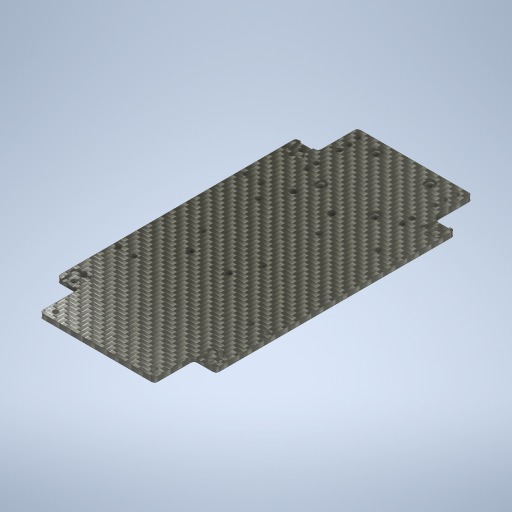
# Autodesk Inventor part: FootSoleFrame
Saved by Autodesk Inventor 2024.2 (Build 282272000, 272)
## iProperties
Created: 2024-01-07
Part Number: FootSoleFrame
Material: CFRP
Document SubType Name: Modeling
Designer: Masato Kubotera
Density: 1.43 g/cm^3
Appearance: Carbon Fiber 1
Mass: 79.1828 g
Surface Area: 392.308 cm^2
Volume: 55.3726 cm^3
Vendor: ALLPCB
Author: Masato Kubotera
Autodesk Inventor part; units mm, degrees
ref_plane "YZ Plane" through (0, 0, 0) normal (1, 0, 0) x (0, 1, 0)
ref_plane "XZ Plane" through (0, 0, 0) normal (0, 1, 0) x (-1, 0, 0)
ref_plane "XY Plane" through (0, 0, 0) normal (0, 0, 1) x (1, 0, 0)
sketch "Sketch1" plane through (0, 0, 0) normal (0, 0, 1) x (1, 0, 0)
  line L0 (-100, 59.95) -> (100, 59.95)
  line L1 (100, 59.95) -> (100, -40.05)
  line L2 (100, -40.05) -> (-100, -40.05)
  line L3 (-100, -40.05) -> (-100, 59.95)
  line L4 (-100, 59.95) -> (100, -40.05) construction
  line L5 (100, 59.95) -> (-100, -40.05) construction
  line L6 (0, -40.05) -> (0, 59.95) construction
  line L7 (-100, 9.95) -> (100, 9.95) construction
  line L8 (-100, 0) -> (100, 0) construction
  line L9 (-44, -22.5) -> (18, -22.5) construction
  line L10 (18, -22.5) -> (18, 22.5) construction
  line L11 (18, 22.5) -> (-44, 22.5) construction
  line L12 (-44, 22.5) -> (-44, -22.5) construction
  line L13 (-44, -22.5) -> (18, 22.5) construction
  line L14 (18, -22.5) -> (-44, 22.5) construction
  line L15 (13, -22.5) -> (13, 22.5) construction
  line L16 (4.5, -19) -> (4.5, 19) construction
  line L17 (-13, -22.5) -> (-13, 22.5) construction
  line L18 (-39, -22.5) -> (-39, 22.5) construction
  line L19 (100, 46.05) -> (75.15, 46.05)
  line L20 (75.15, 46.05) -> (75.15, 59.95)
  line L21 (65.2, 49.05) -> (97, 49.05) construction
  line L22 (97, 49.05) -> (97, 56.95) construction
  line L23 (97, 56.95) -> (65.2, 56.95) construction
  line L24 (65.2, 56.95) -> (65.2, 49.05) construction
  line L25 (65.2, 49.05) -> (97, 56.95) construction
  line L26 (97, 49.05) -> (65.2, 56.95) construction
  line L27 (65.2, 53) -> (97, 53) construction
  line L28 (81.1, 49.05) -> (81.1, 56.95) construction
  circle A0 centre (71.55, 53) radius 1.6 construction
  circle A1 centre (65.2, 53) radius 1.6 construction
  line L29 (100, -26.15) -> (75.15, -26.15)
  line L30 (75.15, -26.15) -> (75.15, -40.05)
  line L31 (-100, 46.05) -> (-75.15, 46.05)
  line L32 (-75.15, 46.05) -> (-75.15, 59.95)
  line L33 (-75.15, -26.15) -> (-75.15, -40.05)
  line L34 (-100, -26.15) -> (-75.15, -26.15)
  line L35 (13, -12) -> (18, -12) construction
  line L36 (13, 12) -> (18, 12) construction
  circle A2 centre (95, 41.05) radius 5 construction
  circle A3 centre (95, 41.05) radius 2 construction
  circle A4 centre (95, -21.15) radius 5 construction
  circle A5 centre (95, -21.15) radius 2 construction
  circle A6 centre (-95, 41.05) radius 5 construction
  circle A7 centre (-95, 41.05) radius 2 construction
  circle A8 centre (-95, -21.15) radius 2 construction
  circle A9 centre (-95, -21.15) radius 5 construction
  line L37 (-53.66, -15.05) -> (-96.84, -15.05) construction
  line L38 (-96.84, -15.05) -> (-96.84, 34.95) construction
  line L39 (-96.84, 34.95) -> (-53.66, 34.95) construction
  line L40 (-53.66, 34.95) -> (-53.66, -15.05) construction
  line L41 (-53.66, -15.05) -> (-96.84, 34.95) construction
  line L42 (-96.84, -15.05) -> (-53.66, 34.95) construction
  line L43 (-75.25, -15.05) -> (-75.25, 34.95) construction
  line L44 (-57.91, -7.05) -> (-92.59, -7.05) construction
  line L45 (-92.59, -7.05) -> (-92.59, 26.95) construction
  line L46 (-92.59, 26.95) -> (-57.91, 26.95) construction
  line L47 (-57.91, 26.95) -> (-57.91, -7.05) construction
  line L48 (-57.91, -7.05) -> (-92.59, 26.95) construction
  line L49 (-92.59, -7.05) -> (-57.91, 26.95) construction
  line L50 (22, 23.5) -> (-50.5, 23.5) construction
  line L51 (-50.5, 23.5) -> (-50.5, -23.5) construction
  line L52 (-50.5, -23.5) -> (22, -23.5) construction
  line L53 (22, -23.5) -> (22, 23.5) construction
  line L54 (22, 23.5) -> (-50.5, -23.5) construction
  line L55 (-50.5, 23.5) -> (22, -23.5) construction
  line L56 (75.15, 49) -> (65.2, 49)
  line L57 (65.2, 49) -> (65.2, 57)
  line L58 (65.2, 57) -> (75.15, 57)
  line L59 (75.15, -29.1) -> (65.2, -29.1)
  line L60 (65.2, -29.1) -> (65.2, -37.1)
  line L61 (65.2, -37.1) -> (75.15, -37.1)
  line L62 (-75.15, 49) -> (-65.2, 49)
  line L63 (-65.2, 49) -> (-65.2, 57)
  line L64 (-65.2, 57) -> (-75.15, 57)
  line L65 (-75.15, -29.1) -> (-65.2, -29.1)
  line L66 (-65.2, -29.1) -> (-65.2, -37.1)
  line L67 (-65.2, -37.1) -> (-75.15, -37.1)
  arc A10 (69.2, 57) -> (65.2, 57) centre (67.2, 57) ccw
  arc A11 (65.2, 49) -> (69.2, 49) centre (67.2, 49) ccw
  arc A12 (65.2, -37.1) -> (69.2, -37.1) centre (67.2, -37.1) ccw
  arc A13 (69.2, -29.1) -> (65.2, -29.1) centre (67.2, -29.1) ccw
  arc A14 (-65.2, 57) -> (-69.2, 57) centre (-67.2, 57) ccw
  arc A15 (-69.2, 49) -> (-65.2, 49) centre (-67.2, 49) ccw
  arc A16 (-65.2, -29.1) -> (-69.2, -29.1) centre (-67.2, -29.1) ccw
  arc A17 (-69.2, -37.1) -> (-65.2, -37.1) centre (-67.2, -37.1) ccw
  line L68 (100, -31.775) -> (-100, -31.775) construction
  line L69 (-82.41, -20.05) -> (-88.41, -20.05) construction
  line L70 (-40, -36.775) -> (-40, -26.775) construction
  circle A18 centre (54.6684, 54.95) radius 5 construction
  circle A19 centre (-88.41, -20.05) radius 1.6 construction
  point P0 (0, 0)
  point P1 (0, 9.95)
  point P2 (-13, 0)
  point P3 (-30.5, -19)
  point P4 (-30.5, 19)
  point P5 (81.1, 53)
  point P6 (90.65, 53)
  point P7 (-75.15, 59.95)
  point P8 (-75.15, -40.05)
  point P9 (75.15, -40.05)
  point P10 (65.2, -33.1)
  point P11 (71.55, -33.1)
  point P12 (-65.2, 53)
  point P13 (-71.55, 53)
  point P14 (-65.2, -33.1)
  point P15 (-71.55, -33.1)
  point P16 (19.5, -12)
  point P17 (19.5, 12)
  point P18 (-45.5, -12)
  point P19 (-45.5, 12)
  point P20 (-75.25, 9.95)
  point P21 (-14.25, 0)
  point P22 (75.15, -37.1)
  point P23 (75.15, -29.1)
  point P24 (-65.2, -30.2522)
  point P25 (-65.2, -29.1)
  point P26 (-65.2, -29.1)
  point P27 (-69.2, -29.1)
  point P28 (-69.2, -37.1)
  point P29 (-65.2, -37.1)
  point P30 (-65.2, -37.1)
  point P31 (-65.2, -35.9478)
  point P32 (-65.2, 57)
  point P33 (-65.2, 55.8478)
  point P34 (-69.2, 57)
  point P35 (-69.2, 49)
  point P36 (-65.2, 50.1522)
  point P37 (65.2, 50.1522)
  point P38 (69.2, 49)
  point P39 (69.2, -29.1)
  point P40 (65.2, -30.2522)
  point P41 (65.2, -35.9478)
  point P42 (69.2, -37.1)
  point P43 (-85.41, -20.05)
  point P44 (-40, -31.775)
  point P45 (-68.09, -20.05)
  point P46 (-62.09, -20.05)
  point P47 (-82.41, 39.95)
  point P48 (-88.41, 39.95)
  point P49 (-68.09, 39.95)
  point P50 (-62.09, 39.95)
  point P51 (40, -36.775)
  point P52 (40, -26.775)
  point P53 (-40, 56.675)
  point P54 (-40, 46.675)
  point P55 (40, 46.675)
  point P56 (40, 56.675)
  dimension "d0" = 200
  dimension "d1" = 100
  dimension "d2" = 62
  dimension "d3" = 45
  dimension "d4" = 80.1
  dimension "d5" = 5
  dimension "d7" = 38
  dimension "d8" = 35
  dimension "d9" = 31.8
  dimension "d10" = 7.9
  dimension "d11" = 19.1
  dimension "d12" = 3
  dimension "d13" = 3
  dimension "d14" = 3.2
  dimension "d15" = 2
  dimension "d27" = 87
  dimension "d28" = 24
  dimension "d29" = 1.5
  dimension "d37" = 6.95
  dimension "d38" = 4.5
  dimension "d39" = 4
  dimension "d40" = 10
  dimension "d41" = 43.18
  dimension "d42" = 50
  dimension "d43" = 8.5
  dimension "d44" = 16
  dimension "d45" = 6.5
  dimension "d46" = 4
  dimension "d47" = 1
  dimension "d48" = 0.05
  dimension "d51" = 2
  dimension "d62" = 6
  dimension "d63" = 5
  dimension "d64" = 20.32
  dimension "d65" = 10
  dimension "d67" = 80
  constraints: 142 end point, 78 symmetric about line, 27 midpoint, 23 point on line, 20 centre point, 19 coincident, 16 point on circle, 13 parallel, 12 horizontal, 6 perpendicular, 5 vertical, 4 tangent, 3 equal radius, 1 collinear, 18 other
  measures "d0" distance of L1.end L2.end
  measures "d1" distance of L0.end L1.end
  measures "d2" distance of L11.end L10.end
  measures "d3" distance of L10.end L9.end
  measures "d4" diameter of L2 L8
  measures "d5" distance between parallel lines of L10 L15
  measures "d7" distance of L16.end L16.start
  measures "d8" distance of point (4.5, 19) point (-30.5, 19)
  measures "d9" distance of L23.end L22.end
  measures "d10" distance of L22.end L21.end
  measures "d11" distance of point (71.55, 53) point (90.65, 53)
  measures "d12" distance between parallel lines of L0 L23
  measures "d13" distance between parallel lines of L1 L22
  measures "d14" diameter of A0
  measures "d15" distance edge to line of A0 L20
  measures "d27" distance between parallel lines of L3 L17
  measures "d28" distance between parallel lines of L36 L35
  measures "d29" distance from line of point (19.5, 12) L10
  measures "d37" distance between parallel lines of L0 L27
  measures "d38" distance between parallel lines of L16 L6
  measures "d39" diameter of A3
  measures "d40" diameter of A2
  measures "d41" distance of L38.end L39.end
  measures "d42" distance of L37.end L38.end
  measures "d43" diameter of L40 L47
  measures "d44" diameter of L39 L46
  measures "d45" distance between parallel lines of L51 L12
  measures "d46" distance between parallel lines of L53 L10
  measures "d47" distance between parallel lines of L52 L9
  measures "d48" distance between parallel lines of L56 L21
  measures "d51" radius of A10
  measures "d62" distance of L69.end L69.start
  measures "d63" distance between parallel lines of L37 L69
  measures "d64" diameter of point (-85.41, -20.05) L43
  measures "d65" distance of L70.end L70.start
  measures "d67" distance of L70.start point (40, -36.775)
extrude "Extrusion1" add sketch "Sketch1" against normal blind 3 contours L0 L20 L58 A10 L57 A11 L56 L19 L1 L29 L30 L59 A13 L60 A12 L61 L2 L33 L67 A17 L66 A16 L65 L34 L3 L31 L32 L62 A15 L63 A14 L64 | L64 L63 L62 L32 | L20 L56 L57 L58 | A14 L64 | L58 A10 | L62 A15 | L65 L66 L67 L33 | A11 L56 | A16 L65 | L61 L60 L59 L30 | L67 A17 | A12 L61 | L59 A13
extrude "Extrusion2" cut sketch "Sketch1" against normal blind 1 contours L64 L63 L62 L32 | L20 L56 L57 L58 | A14 L64 | L58 A10 | L62 A15 | L65 L66 L67 L33 | A11 L56 | A16 L65 | L61 L60 L59 L30 | L67 A17 | A12 L61 | L59 A13
hole "Phi3.2" at (4.5, -19, 0) at (4.5, 19, 0) at (-30.5, -19, 0) at (-30.5, 19, 0) at (65.2, 53, 0) at (71.55, 53, 0) at (90.65, 53, 0) at (65.2, -33.1, 0) at (71.55, -33.1, 0) at (-71.55, -33.1, 0) at (-65.2, -33.1, 0) at (-65.2, 53, 0) at (-71.55, 53, 0) at (95, -21.15, 0) at (95, 41.05, 0) at (-95, 41.05, 0) at (-95, -21.15, 0) at (-88.41, -20.05, 0) at (-82.41, -20.05, 0) at (-40, -26.775, 0) at (-40, -36.775, 0) at (-68.09, -20.05, 0) at (-62.09, -20.05, 0) at (-88.41, 39.95, 0) at (-82.41, 39.95, 0) at (-68.09, 39.95, 0) at (-62.09, 39.95, 0) at (40, -26.775, 0) at (40, -36.775, 0) at (40, 46.675, 0) at (40, 56.675, 0) at (-40, 56.675, 0) at (-40, 46.675, 0) direction (0, 0, -1) diameter 3.2 end through all
hole "Phi4.0" at (19.5, -12, 0) at (19.5, 12, 0) at (-45.5, -12, 0) at (-45.5, 12, 0) direction (0, 0, -1) diameter 4 end through all
hole "Phi6.5-3.2" at (-57.91, -7.05, 0) at (-57.91, 26.95, 0) at (-92.59, 26.95, 0) at (-92.59, -7.05, 0) direction (0, 0, -1) diameter 3.2 end through all counterbore diameter 6.5 counterbore depth 1
fillet "R2" radius 2 12 edges at (100, 46.05, -1.5) (100, -26.15, -1.5) (75.15, -40.05, -1.5) (75.15, -26.15, -1.5) (75.15, 46.05, -1.5) (75.15, 59.95, -1.5) (-75.15, 59.95, -1.5) (-75.15, 46.05, -1.5) (-100, 46.05, -1.5) (-100, -26.15, -1.5) (-75.15, -26.15, -1.5) (-75.15, -40.05, -1.5)
equation "\"d13\" = d12"
equation "\"d19\" = d14"
body "Solid1"
